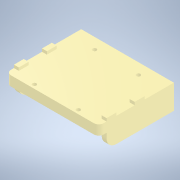
# Autodesk Inventor part: Attaching Point
Saved by Autodesk Inventor 2022 (Build 260153000, 153)
## iProperties
Created: 2021-06-18
Part Number: Attaching Point
Material: Nylon 6/6
Document SubType Name: Modeling
Designer: benka
Density: 1.13 g/cm^3
Appearance: Nylon 6
Author: benka
Autodesk Inventor part; units mm, degrees
ref_plane "YZ Plane" through (0, 0, 0) normal (1, 0, 0) x (0, 1, 0)
ref_plane "XZ Plane" through (0, 0, 0) normal (0, 1, 0) x (-1, 0, 0)
ref_plane "XY Plane" through (0, 0, 0) normal (0, 0, 1) x (1, 0, 0)
sketch "Sketch1" plane through (0, 0, 0) normal (0, 0, 1) x (1, 0, 0)
  line L0 (42.5, -5) -> (47.4999, -5)
  line L1 (42.5, -10) -> (-42.5, -10)
  line L2 (42.5, -10) -> (42.5, -5)
  line L3 (-42.5, -10) -> (-42.5, -4.9999)
  line L4 (-42.5, -4.9999) -> (-47.5001, -5)
  line L5 (-42.5001, 10) -> (-22.5001, 10)
  line L6 (-42.5001, 10) -> (-42.5001, 5)
  line L7 (42.4999, 10) -> (42.4999, 5)
  line L8 (-42.5001, 5) -> (-47.5001, 5)
  line L9 (42.4999, 5) -> (47.4999, 5)
  line L10 (22.4999, 10) -> (42.4999, 10)
  line L11 (-22.5001, 5) -> (-22.5001, 10)
  line L12 (-22.5001, 5) -> (22.4999, 5)
  line L13 (22.4999, 5) -> (22.4999, 10)
  circle A0 centre (30, 0) radius 2
  circle A1 centre (-30, 0) radius 2
  line L14 (-47.5001, -5) -> (-47.5001, 5)
  line L15 (47.4999, 5) -> (47.4999, -5)
  point P0 (0, 0)
  point P1 (-34.7671, -4.6223)
  dimension "d0" = 4
  dimension "d12" = 30
  dimension "d13" = 4
  dimension "d14" = 30
  dimension "d15" = 20
  dimension "d16" = 20
  dimension "d17" = 42.5
  dimension "d18" = 42.5
  dimension "d21" = 45
  dimension "d32" = 5
  dimension "d33" = 5
  constraints: 32 end point, 4 vertical, 2 centre point, 1 coincident, 2 other
  measures "d0" diameter of A0
  measures "d12" distance of A0.centre point (0, 0)
  measures "d13" diameter of A1
  measures "d14" distance of A1.centre point (0, 0)
  measures "d15" distance between parallel lines of L11 L6
  measures "d16" distance between parallel lines of L7 L13
  measures "d17" distance from line of L3 point (0, 0)
  measures "d18" distance from line of L2 point (0, 0)
  measures "d21" distance between parallel lines of L13 L11
  measures "d32" distance of L6.end L8.end
  measures "d33" distance of L7.end L9.end
extrude "Leap AP" add sketch "Sketch1" along normal blind 5
sketch "Sketch2" plane through (-22.5001, 5, 0) normal (0, 1, 0) x (1, 0, 0)
  line L0 (-25, -56) -> (-20, -56)
  line L1 (70, -56) -> (65, -56)
  line L2 (-20, -56) -> (-20, -69)
  line L3 (-20, -69) -> (-25, -69)
  line L4 (-25, -69) -> (-25, -72)
  line L5 (65, -56) -> (65, -69)
  line L6 (65, -69) -> (70, -69)
  line L7 (70, -69) -> (70, -72)
  line L8 (65, -77) -> (-20, -77)
  line L9 (0, -5) -> (0, 0)
  arc A0 (-25, -72) -> (-20, -77) centre (-20, -72) ccw
  arc A1 (65, -77) -> (70, -72) centre (65, -72) ccw
  line L10 (0, -5) -> (-25, -5)
  line L11 (45, 0) -> (0, 0) projected
  line L12 (45, 0) -> (45, -5)
  circle A2 centre (0, -73) radius 2
  circle A3 centre (45, -73) radius 2
  line L13 (-25, -56) -> (-25, -5)
  line L14 (70, -56) -> (70, -5)
  circle A4 centre (0, -11.3502) radius 2
  circle A5 centre (45, -11.3502) radius 2
  line L15 (45, -5) -> (70, -5)
  point P0 (-25, -77)
  point P1 (70, -77)
  point P2 (69.9999, -5)
  point P3 (11.4357, -9.3722)
  dimension "d52" = 13
  dimension "d54" = 8
  dimension "d55" = 5
  dimension "d56" = 5
  dimension "d74" = 4
  dimension "d75" = 4
  dimension "d76" = 4
  dimension "d77" = 4
  dimension "d78" = 25
  dimension "d79" = 25
  dimension "d83" = 51
  dimension "d84" = 4
  dimension "d85" = 4
  constraints: 30 end point, 6 centre point, 5 collinear, 5 perpendicular, 5 point on line, 4 point on circle, 4 tangent, 1 horizontal, 1 parallel, 1 other
  measures "d52" distance of L0.end L2.end
  measures "d54" distance of L3.end point (-25, -77)
  measures "d55" radius of A0
  measures "d56" radius of A1
  measures "d74" diameter of A2
  measures "d75" diameter of A3
  measures "d76" distance from line of A2.centre L8
  measures "d77" distance from line of L8 A3.centre
  measures "d78" distance from line of L4 A2.centre
  measures "d79" distance from line of L7 A3.centre
  measures "d83" distance of L0.start L10.end
  measures "d84" diameter of A4
  measures "d85" diameter of A5
extrude "Leap Base" add sketch "Sketch2" along normal blind 5
sketch "Sketch3" plane through (-42.5001, 5, 0) normal (-1, 0, 0) x (0, 0, 1)
  line L0 (0, -9.9999) -> (5, -9.9999) projected
  line L1 (0, -9.9999) -> (0, -15) projected
  line L2 (0, -15) -> (5, -15) projected
  line L3 (0, 0) -> (5, 0) projected
  line L4 (5, -9.9999) -> (5, 0)
  line L5 (5, -15) -> (59, -15)
  line L6 (0, 0) -> (0, 5) projected
  line L7 (69, 5) -> (69, 13)
  line L8 (69, 5) -> (69, -5)
  arc A0 (59, -15) -> (69, -5) centre (59, -5) ccw
  line L9 (69, 13) -> (58.8965, 13)
  line L10 (58.8965, 13) -> (58.8965, 5)
  line L11 (40.1783, 5) -> (40.1783, 13)
  line L12 (40.1783, 13) -> (30.0747, 13)
  line L13 (30.0747, 13) -> (30.0747, 5)
  line L14 (0, 5) -> (30.0747, 5)
  line L15 (40.1783, 5) -> (58.8965, 5)
  point P0 (69, -15)
  point P1 (8.1162, -2.0146)
  dimension "d72" = 10
  dimension "d86" = 8
  constraints: 22 end point, 4 perpendicular, 3 horizontal, 3 vertical, 2 collinear, 2 point on circle, 2 point on line, 2 tangent, 1 centre point, 1 other
  measures "d72" radius of A0
  measures "d86" distance of L7.start L7.end
extrude "2x Leap Side" add sketch "Sketch3" along normal blind 5
sketch "Sketch4" plane through (42.4999, 5, 0) normal (1, 0, 0) x (0, 0, -1)
  line L0 (0, 5) -> (0, -15) projected
  line L1 (0, -15) -> (-59, -15) projected
  arc A0 (-69, -5) -> (-59, -15) centre (-59, -5) ccw projected
  line L2 (-69, -5) -> (-69, 0) projected
  line L3 (-69, 0) -> (-72, 0) projected
  line L4 (-72, 0) -> (-72, 5) projected
  line L5 (-69, 5) -> (-72, 5) projected
  line L6 (-69, 5) -> (-69, 13) projected
  line L7 (-69, 13) -> (-58.8965, 13) projected
  line L8 (-58.8965, 13) -> (-58.8965, 5) projected
  line L9 (-30.0747, 5) -> (0, 5) projected
  line L10 (-40.1783, 5) -> (-58.8965, 5) projected
  line L11 (-40.1783, 5) -> (-40.1783, 13) projected
  line L12 (-40.1783, 13) -> (-30.0747, 13) projected
  line L13 (-30.0747, 13) -> (-30.0747, 5) projected
extrude "Extrusion4" add sketch "Sketch4" along normal blind 5
sketch "Sketch5" plane through (-47.5001, 10, 0) normal (0, 1, 0) x (1, 0, 0)
  line L0 (5, -58.8965) -> (0, -58.8965) projected
  line L1 (5, -69) -> (5, -58.8965) projected
  line L2 (5, -69) -> (0, -69) projected
  line L3 (0, -69) -> (0, -72) projected
  arc A0 (0, -72) -> (5, -77) centre (5, -72) ccw projected
  line L4 (5, -77) -> (90, -77) projected
  arc A1 (90, -77) -> (95, -72) centre (90, -72) ccw projected
  circle A2 centre (25, -73) radius 2 projected
  circle A3 centre (70, -73) radius 2 projected
  line L5 (0, 0) -> (95, 0) projected
  line L6 (0, -30.0747) -> (0, 0) projected
  line L7 (95, -40.1783) -> (95, -58.8965) projected
  line L8 (95, -30.0747) -> (95, 0) projected
  line L9 (0, -40.1783) -> (0, -58.8965) projected
  line L10 (90, -58.8965) -> (90, -69) projected
  line L11 (90, -58.8965) -> (95, -58.8965) projected
  line L12 (5, -30.0747) -> (0, -30.0747) projected
  line L13 (5, -40.1783) -> (5, -30.0747) projected
  line L14 (5, -40.1783) -> (0, -40.1783) projected
  line L15 (90, -40.1783) -> (95, -40.1783) projected
  line L16 (90, -30.0747) -> (90, -40.1783) projected
  line L17 (90, -30.0747) -> (95, -30.0747) projected
  line L18 (90, -69) -> (95, -69) projected
  line L19 (95, -72) -> (95, -69) projected
  circle A4 centre (25, -11.3502) radius 2 projected
  circle A5 centre (70, -11.3502) radius 2 projected
  point P0 (31.9525, -5.2817)
  constraints: 1 other
extrude "Leap Top Base" add sketch "Sketch5" along normal blind 5
body "Solid1"
